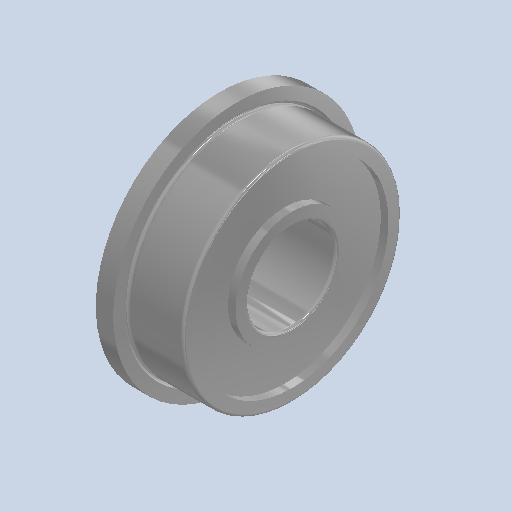
# Autodesk Inventor part: FL696ZZ_CPY2
Saved by Autodesk Inventor 2024 (Build 280153000, 153)
## iProperties
Part Number: FL696ZZ_CPY2
Material: 一般
Catalog Web Link: www.cadenas.de
Description: FL6 _ _ ZZ, FL6 _ _ AZZ, SFL6 _ _ ZZ, SFL6 _ _ AZZ, MFL1 _ _ ZZ, SMFL1 _ _ ZZ-Flanged Ball Bearings (Small Diameter, Deep Groove) - Double Shield Type
Vendor: MISUMI
Document SubType Name: Modeling
Designer: tanoue_kota
Manufacturer: MISUMI
Mass: 0.70407 g
Surface Area: 8.21849 cm^2
Volume: 0.70407 cm^3
Density: 1 g/cm^3
Appearance: アルミニウム - つや出し
Category: PARTsolutions
Company: MISUMI
Title: FL696ZZ
Author: Cadenas PARTsolutions
Comments: Flanged Ball Bearings (Small Diameter, Deep Groove) - Double Shield Type
PSOL_IDENT_0: {$CADENAS_DATA\23d-libs\misumi\metric\12_bearing_holders\sfl608zz.prj},229 {VTYP=3D},{NB=FL696ZZ},{L
PSOL_IDENT_1: INA=FL696ZZ},{NN=FL6 _ _ ZZ, FL6 _ _ AZZ, SFL6 _ _ ZZ, SFL6 _ _ AZZ, MFL1 _ _ ZZ, SMFL1 _ _ ZZ},{DAT
PSOL_IDENT_2: E=09.09.2019 15:26:56},{GEOMDATE=16.08.2017 04:27:24},{VERSION=},{LINEID=110},{WBVAR=MAT},{WBNUMERIC=
PSOL_IDENT_3: }  {NB=FL696ZZ},{LINA=FL696ZZ},{KT=DUMMY},{PN=FL696ZZ},{MAT=},{MAT1= '', '52100 Bearing Steel', 'S',
PSOL_IDENT_4: '440C Stainless Steel'},{BN=696ZZ},{DD=6.0},{AA=3.9525},{BB=0.9000},{C1=0.9000},{D=15},{B=5.0},{D1=
PSOL_IDENT_5: 17.0},{C=1.2},{RR=0.20},{CR=1350},{COR=530},{CRS=1350},{CRSS=1139},{CORS=530},{CORSS=418},{DS=7.60},
PSOL_IDENT_6: {R=0.20},{MASS=4.3},{MAT11=1},{MMMM=}
NB: FL696ZZ
NN: FL6 _ _ ZZ, FL6 _ _ AZZ, SFL6 _ _ ZZ, SFL6 _ _ AZZ, MFL1 _ _ ZZ, SMFL1 _ _ ZZ
NT: Flanged Ball Bearings (Small Diameter, Deep Groove) - Double Shield Type
NBSYN: $PN.
LINA: FL696ZZ
CATALOG: Misumi
PN: FL696ZZ
MAT: 52100 Bearing Steel
BN: 696ZZ
DD: 6
D: 15
B: 5
D1: 0
C: 1.2
RR: 0.2
CR: 1350
COR: 530
DS: 7.6
R: 0.2
MASS: 4.3
SUPPLIER: MISUMI
ARTICLENO: FL696ZZ
BOMINFO: FL696ZZ
CREATOR: CADENAS GmbH
Autodesk Inventor part; units mm, degrees
sketch "Sketch_1" plane through (0, 0, 0) normal (0, 0, 1) x (1, 0, 0)
  line L0 (15, 0) -> (-15, 0)
  arc A0 (0, 3.2) -> (0.2, 3) centre (0.2, 3.2) ccw
  line L1 (0.2, 3) -> (4.8, 3)
  arc A1 (4.8, 3) -> (5, 3.2) centre (4.8, 3.2) ccw
  line L2 (5, 3.2) -> (5, 3.9)
  line L3 (5, 3.9) -> (4.4763, 3.9)
  line L4 (4.4763, 3.9) -> (4.4763, 6.6)
  line L5 (4.4763, 6.6) -> (5, 6.6)
  line L6 (5, 6.6) -> (5, 8.5)
  line L7 (5, 8.5) -> (3.8, 8.5)
  line L8 (3.8, 8.5) -> (3.8, 7.7)
  arc A2 (3.6, 7.5) -> (3.8, 7.7) centre (3.8, 7.5) ccw
  line L9 (3.6, 7.5) -> (0.2, 7.5)
  arc A3 (0.2, 7.5) -> (0, 7.3) centre (0.2, 7.3) ccw
  line L10 (0, 7.3) -> (0, 6.6)
  line L11 (0, 6.6) -> (0.5238, 6.6)
  line L12 (0.5238, 6.6) -> (0.5238, 3.9)
  line L13 (0.5238, 3.9) -> (0, 3.9)
  line L14 (0, 3.9) -> (0, 3.2)
  constraints: 30 end point, 8 point on circle, 4 centre point
revolve "Revolution1" add sketch "Sketch_1" angle 360 about axis through (15, 0, 0) along (1, 0, 0)
ref_plane "to_housing_XY" through (0, 0, 0) normal (1, 0, 0) x (0, 0, -1)
ref_plane "to_housing_YZ" through (0, 0, 0) normal (0, 0, -1) x (0, 1, 0)
ref_plane "to_housing_ZX" through (0, 0, 0) normal (0, 1, 0) x (1, 0, 0)
body "Solid1"
